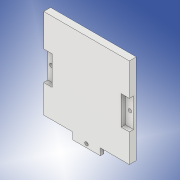
# Autodesk Inventor part: TC008
Saved by Autodesk Inventor 2017 SP1 (Build 210196100, 196)
## iProperties
Created: 2017-08-15
Part Number: TC008
Material: ABS Plastic
Document SubType Name: Modeling
Designer: Zach
Density: 1.06 g/cm^3
Appearance: CR White
Author: Zach
Autodesk Inventor part; units mm, degrees
ref_plane "YZ Plane" through (0, 0, 0) normal (1, 0, 0) x (0, 1, 0)
ref_plane "XZ Plane" through (0, 0, 0) normal (0, 1, 0) x (-1, 0, 0)
ref_plane "XY Plane" through (0, 0, 0) normal (0, 0, 1) x (1, 0, 0)
sketch "Sketch1" plane through (0, 0, 0) normal (0, 0, 1) x (1, 0, 0)
  line L0 (0, 0) -> (124, 0)
  line L1 (124, 0) -> (124, 124)
  line L2 (124, 124) -> (0, 124)
  line L3 (0, 124) -> (0, 0)
  circle A0 centre (5, 62) radius 2.5
  circle A1 centre (119, 62) radius 2.5
  point P0 (124, 62)
  point P1 (0, 62)
  dimension "d0" = 124
  dimension "d1" = 124
  dimension "d2" = 5
  dimension "d3" = 5
  dimension "d4" = 5
  dimension "d5" = 5
  constraints: 8 end point, 2 centre point, 2 horizontal alignment, 2 midpoint, 2 parallel, 1 horizontal, 1 perpendicular
  measures "d0" distance of L2.end L1.end
  measures "d1" distance of L1.end L0.end
  measures "d2" diameter of A0
  measures "d3" diameter of A1
  measures "d4" distance from line of L3 A0.centre
  measures "d5" distance from line of L1 A1.centre
extrude "Extrusion1" add sketch "Sketch1" along normal blind 10
sketch "Sketch2" plane through (0, 0, 10) normal (0, 0, 1) x (1, 0, 0)
  line L0 (42, 0) -> (82, 0)
  line L1 (82, 0) -> (82, -10)
  line L2 (82, -10) -> (42, -10)
  line L3 (42, -10) -> (42, 0)
  circle A0 centre (62, -5) radius 2.5
  line L4 (0, 0) -> (124, 0) projected
  point P0 (82, -5)
  point P1 (62, -10)
  point P2 (62, 0)
  dimension "d8" = 40
  dimension "d9" = 10
  dimension "d10" = 5
  constraints: 8 end point, 3 midpoint, 2 parallel, 2 vertical alignment, 1 centre point, 1 horizontal, 1 horizontal alignment, 1 perpendicular, 1 point on line
  measures "d8" distance of L1.end L2.end
  measures "d9" distance of L0.end L1.end
  measures "d10" diameter of A0
extrude "Extrusion2" add sketch "Sketch2" against normal blind 5
sketch "Sketch3" plane through (0, 0, 10) normal (0, 0, 1) x (1, 0, 0)
  line L0 (0, 124) -> (0, 0) projected
  line L1 (0, 83) -> (12, 83)
  line L2 (12, 83) -> (12, 41)
  line L3 (12, 41) -> (0, 41)
  line L4 (0, 41) -> (0, 83)
  line L5 (124, 0) -> (124, 124) projected
  line L6 (124, 41) -> (112, 41)
  line L7 (112, 41) -> (112, 83)
  line L8 (112, 83) -> (124, 83)
  line L9 (124, 83) -> (124, 41)
  point P0 (124, 62)
  point P1 (124, 62)
  dimension "d13" = 12
  dimension "d14" = 42
  dimension "d15" = 12
  dimension "d16" = 42
  constraints: 16 end point, 4 parallel, 3 point on line, 2 horizontal, 2 midpoint, 2 perpendicular, 1 coincident
  measures "d13" distance of L2.end L3.end
  measures "d14" distance of L1.end L2.end
  measures "d15" distance of L7.end L8.end
  measures "d16" distance of L6.end L7.end
extrude "Extrusion3" cut sketch "Sketch3" against normal blind 6
sketch "Sketch4" plane through (0, 0, 10) normal (0, 0, 1) x (1, 0, 0)
  line L0 (0, 124) -> (0, 0) projected
  line L1 (0, 124) -> (124, 124)
  line L2 (124, 124) -> (124, 130)
  line L3 (124, 130) -> (0, 130)
  line L4 (0, 130) -> (0, 124)
  dimension "d19" = 6
  constraints: 8 end point, 2 parallel, 1 coincident, 1 horizontal, 1 perpendicular
  measures "d19" distance of L2.end L1.end
extrude "Extrusion4" add sketch "Sketch4" against normal blind 10
body "Solid1"
